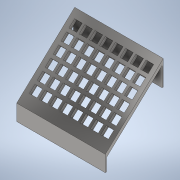
# Autodesk Inventor part: Rejilla_12x12mm
Saved by Autodesk Inventor 2021 (Build 250183000, 183)
## iProperties
Created: 2021-06-27
Part Number: Rejilla_12x12mm
Material: Acero inoxidable
Document SubType Name: Modeling
Designer: artur
Density: 8 g/cm^3
Appearance: Acero - Pulido
Author: artur
Autodesk Inventor part; units mm, degrees
ref_plane "YZ Plane" through (0, 0, 0) normal (1, 0, 0) x (0, 1, 0)
ref_plane "XZ Plane" through (0, 0, 0) normal (0, 1, 0) x (-1, 0, 0)
ref_plane "XY Plane" through (0, 0, 0) normal (0, 0, 1) x (1, 0, 0)
sketch "Boceto3" plane through (0, 0, 0) normal (0, 0, 1) x (1, 0, 0)
  line L0 (118.929, 0) -> (171.1141, 0) construction
  line L1 (0, 0) -> (-79.0081, 0) construction
  line L2 (0, 0) -> (91, 84.6517)
  line L3 (0, 0) -> (0, -24.9684)
  line L4 (0, -24.9684) -> (2, -24.9684)
  line L5 (2, -24.9684) -> (2, -4.9684)
  line L6 (80.5422, 57.5078) -> (86.2007, 57.5078)
  line L7 (91, 84.6517) -> (91, 45.9623)
  line L8 (91, 45.9623) -> (89, 45.9623)
  line L9 (89, 45.9623) -> (89, 75.9623)
  line L10 (2, -4.9684) -> (89, 75.9623)
  dimension "d118" = 137.07
  dimension "d120" = 2
  dimension "d122" = 5
  dimension "d123" = 30
  dimension "d124" = 2
  dimension "d125" = 5
  dimension "d147" = 20
  dimension "d149" = 89
  constraints: 22 end point, 4 horizontal, 2 perpendicular, 2 vertical
  measures "d118" angle of L1 L2
  measures "d120" distance between parallel lines of L5 L3
  measures "d122" distance from line of L2 L9.end
  measures "d123" distance of L8.end L9.end
  measures "d124" distance between parallel lines of L7 L9
  measures "d125" distance from line of L2 L5.end
  measures "d147" distance of L4.end L5.end
  measures "d149" distance between parallel lines of L3 L9
extrude "Extrusión2" add sketch "Boceto3" along normal blind 139
sketch "Boceto7" plane through (0, 0, 0) normal (-0.6811, 0.7322, 0) x (0, 0, 1)
  line L0 (8, 101.2856) -> (20, 101.2856)
  line L1 (20, 101.2856) -> (20, 113.2856)
  line L2 (20, 113.2856) -> (8, 113.2856)
  line L3 (8, 113.2856) -> (8, 101.2856)
  line L4 (0, 124.2856) -> (139, 124.2856) projected
  line L5 (0, 124.2856) -> (0, 0) projected
  line L6 (24, 101.2856) -> (36, 101.2856)
  line L7 (36, 101.2856) -> (36, 113.2856)
  line L8 (36, 113.2856) -> (24, 113.2856)
  line L9 (24, 113.2856) -> (24, 101.2856)
  line L10 (40, 101.2856) -> (52, 101.2856)
  line L11 (52, 101.2856) -> (52, 113.2856)
  line L12 (52, 113.2856) -> (40, 113.2856)
  line L13 (40, 113.2856) -> (40, 101.2856)
  line L14 (56, 101.2856) -> (68, 101.2856)
  line L15 (68, 101.2856) -> (68, 113.2856)
  line L16 (68, 113.2856) -> (56, 113.2856)
  line L17 (56, 113.2856) -> (56, 101.2856)
  line L18 (72, 101.2856) -> (84, 101.2856)
  line L19 (84, 101.2856) -> (84, 113.2856)
  line L20 (84, 113.2856) -> (72, 113.2856)
  line L21 (72, 113.2856) -> (72, 101.2856)
  line L22 (88, 101.2856) -> (100, 101.2856)
  line L23 (100, 101.2856) -> (100, 113.2856)
  line L24 (100, 113.2856) -> (88, 113.2856)
  line L25 (88, 113.2856) -> (88, 101.2856)
  line L26 (104, 101.2856) -> (116, 101.2856)
  line L27 (116, 101.2856) -> (116, 113.2856)
  line L28 (116, 113.2856) -> (104, 113.2856)
  line L29 (104, 113.2856) -> (104, 101.2856)
  line L30 (120, 101.2856) -> (132, 101.2856)
  line L31 (132, 101.2856) -> (132, 113.2856)
  line L32 (132, 113.2856) -> (120, 113.2856)
  line L33 (120, 113.2856) -> (120, 101.2856)
  line L34 (8, 84.2856) -> (20, 84.2856)
  line L35 (8, 96.2856) -> (8, 84.2856)
  line L36 (20, 84.2856) -> (20, 96.2856)
  line L37 (20, 96.2856) -> (8, 96.2856)
  line L38 (24, 96.2856) -> (24, 84.2856)
  line L39 (36, 96.2856) -> (24, 96.2856)
  line L40 (36, 84.2856) -> (36, 96.2856)
  line L41 (24, 84.2856) -> (36, 84.2856)
  line L42 (40, 96.2856) -> (40, 84.2856)
  line L43 (52, 96.2856) -> (40, 96.2856)
  line L44 (40, 84.2856) -> (52, 84.2856)
  line L45 (56, 96.2856) -> (56, 84.2856)
  line L46 (68, 96.2856) -> (56, 96.2856)
  line L47 (56, 84.2856) -> (68, 84.2856)
  line L48 (52, 84.2856) -> (52, 96.2856)
  line L49 (68, 84.2856) -> (68, 96.2856)
  line L50 (72, 96.2856) -> (72, 84.2856)
  line L51 (72, 84.2856) -> (84, 84.2856)
  line L52 (84, 96.2856) -> (72, 96.2856)
  line L53 (84, 84.2856) -> (84, 96.2856)
  line L54 (100, 96.2856) -> (88, 96.2856)
  line L55 (88, 84.2856) -> (100, 84.2856)
  line L56 (88, 96.2856) -> (88, 84.2856)
  line L57 (100, 84.2856) -> (100, 96.2856)
  line L58 (104, 96.2856) -> (104, 84.2856)
  line L59 (116, 96.2856) -> (104, 96.2856)
  line L60 (116, 84.2856) -> (116, 96.2856)
  line L61 (120, 96.2856) -> (120, 84.2856)
  line L62 (132, 84.2856) -> (132, 96.2856)
  line L63 (132, 96.2856) -> (120, 96.2856)
  line L64 (120, 84.2856) -> (132, 84.2856)
  line L65 (104, 84.2856) -> (116, 84.2856)
  line L66 (8, 67.2856) -> (20, 67.2856)
  line L67 (8, 79.2856) -> (8, 67.2856)
  line L68 (20, 67.2856) -> (20, 79.2856)
  line L69 (20, 79.2856) -> (8, 79.2856)
  line L70 (24, 79.2856) -> (24, 67.2856)
  line L71 (36, 79.2856) -> (24, 79.2856)
  line L72 (36, 67.2856) -> (36, 79.2856)
  line L73 (24, 67.2856) -> (36, 67.2856)
  line L74 (40, 79.2856) -> (40, 67.2856)
  line L75 (52, 79.2856) -> (40, 79.2856)
  line L76 (40, 67.2856) -> (52, 67.2856)
  line L77 (56, 79.2856) -> (56, 67.2856)
  line L78 (68, 79.2856) -> (56, 79.2856)
  line L79 (56, 67.2856) -> (68, 67.2856)
  line L80 (52, 67.2856) -> (52, 79.2856)
  line L81 (68, 67.2856) -> (68, 79.2856)
  line L82 (72, 79.2856) -> (72, 67.2856)
  line L83 (72, 67.2856) -> (84, 67.2856)
  line L84 (84, 79.2856) -> (72, 79.2856)
  line L85 (84, 67.2856) -> (84, 79.2856)
  line L86 (100, 79.2856) -> (88, 79.2856)
  line L87 (88, 67.2856) -> (100, 67.2856)
  line L88 (88, 79.2856) -> (88, 67.2856)
  line L89 (100, 67.2856) -> (100, 79.2856)
  line L90 (104, 79.2856) -> (104, 67.2856)
  line L91 (116, 79.2856) -> (104, 79.2856)
  line L92 (116, 67.2856) -> (116, 79.2856)
  line L93 (120, 79.2856) -> (120, 67.2856)
  line L94 (132, 67.2856) -> (132, 79.2856)
  line L95 (132, 79.2856) -> (120, 79.2856)
  line L96 (120, 67.2856) -> (132, 67.2856)
  line L97 (104, 67.2856) -> (116, 67.2856)
  line L98 (8, 50.2856) -> (20, 50.2856)
  line L99 (8, 62.2856) -> (8, 50.2856)
  line L100 (20, 50.2856) -> (20, 62.2856)
  line L101 (20, 62.2856) -> (8, 62.2856)
  line L102 (24, 62.2856) -> (24, 50.2856)
  line L103 (36, 62.2856) -> (24, 62.2856)
  line L104 (36, 50.2856) -> (36, 62.2856)
  line L105 (24, 50.2856) -> (36, 50.2856)
  line L106 (40, 62.2856) -> (40, 50.2856)
  line L107 (52, 62.2856) -> (40, 62.2856)
  line L108 (40, 50.2856) -> (52, 50.2856)
  line L109 (56, 62.2856) -> (56, 50.2856)
  line L110 (68, 62.2856) -> (56, 62.2856)
  line L111 (56, 50.2856) -> (68, 50.2856)
  line L112 (52, 50.2856) -> (52, 62.2856)
  line L113 (68, 50.2856) -> (68, 62.2856)
  line L114 (72, 62.2856) -> (72, 50.2856)
  line L115 (72, 50.2856) -> (84, 50.2856)
  line L116 (84, 62.2856) -> (72, 62.2856)
  line L117 (84, 50.2856) -> (84, 62.2856)
  line L118 (100, 62.2856) -> (88, 62.2856)
  line L119 (88, 50.2856) -> (100, 50.2856)
  line L120 (88, 62.2856) -> (88, 50.2856)
  line L121 (100, 50.2856) -> (100, 62.2856)
  line L122 (104, 62.2856) -> (104, 50.2856)
  line L123 (116, 62.2856) -> (104, 62.2856)
  line L124 (116, 50.2856) -> (116, 62.2856)
  line L125 (120, 62.2856) -> (120, 50.2856)
  line L126 (132, 50.2856) -> (132, 62.2856)
  line L127 (132, 62.2856) -> (120, 62.2856)
  line L128 (120, 50.2856) -> (132, 50.2856)
  line L129 (104, 50.2856) -> (116, 50.2856)
  line L130 (8, 33.2856) -> (20, 33.2856)
  line L131 (8, 45.2856) -> (8, 33.2856)
  line L132 (20, 33.2856) -> (20, 45.2856)
  line L133 (20, 45.2856) -> (8, 45.2856)
  line L134 (24, 45.2856) -> (24, 33.2856)
  line L135 (36, 45.2856) -> (24, 45.2856)
  line L136 (36, 33.2856) -> (36, 45.2856)
  line L137 (24, 33.2856) -> (36, 33.2856)
  line L138 (40, 45.2856) -> (40, 33.2856)
  line L139 (52, 45.2856) -> (40, 45.2856)
  line L140 (40, 33.2856) -> (52, 33.2856)
  line L141 (56, 45.2856) -> (56, 33.2856)
  line L142 (68, 45.2856) -> (56, 45.2856)
  line L143 (56, 33.2856) -> (68, 33.2856)
  line L144 (52, 33.2856) -> (52, 45.2856)
  line L145 (68, 33.2856) -> (68, 45.2856)
  line L146 (72, 45.2856) -> (72, 33.2856)
  line L147 (72, 33.2856) -> (84, 33.2856)
  line L148 (84, 45.2856) -> (72, 45.2856)
  line L149 (84, 33.2856) -> (84, 45.2856)
  line L150 (100, 45.2856) -> (88, 45.2856)
  line L151 (88, 33.2856) -> (100, 33.2856)
  line L152 (88, 45.2856) -> (88, 33.2856)
  line L153 (100, 33.2856) -> (100, 45.2856)
  line L154 (104, 45.2856) -> (104, 33.2856)
  line L155 (116, 45.2856) -> (104, 45.2856)
  line L156 (116, 33.2856) -> (116, 45.2856)
  line L157 (120, 45.2856) -> (120, 33.2856)
  line L158 (132, 33.2856) -> (132, 45.2856)
  line L159 (132, 45.2856) -> (120, 45.2856)
  line L160 (120, 33.2856) -> (132, 33.2856)
  line L161 (104, 33.2856) -> (116, 33.2856)
  line L162 (8, 16.2856) -> (20, 16.2856)
  line L163 (8, 28.2856) -> (8, 16.2856)
  line L164 (20, 16.2856) -> (20, 28.2856)
  line L165 (20, 28.2856) -> (8, 28.2856)
  line L166 (24, 28.2856) -> (24, 16.2856)
  line L167 (36, 28.2856) -> (24, 28.2856)
  line L168 (36, 16.2856) -> (36, 28.2856)
  line L169 (24, 16.2856) -> (36, 16.2856)
  line L170 (40, 28.2856) -> (40, 16.2856)
  line L171 (52, 28.2856) -> (40, 28.2856)
  line L172 (40, 16.2856) -> (52, 16.2856)
  line L173 (56, 28.2856) -> (56, 16.2856)
  line L174 (68, 28.2856) -> (56, 28.2856)
  line L175 (56, 16.2856) -> (68, 16.2856)
  line L176 (52, 16.2856) -> (52, 28.2856)
  line L177 (68, 16.2856) -> (68, 28.2856)
  line L178 (72, 28.2856) -> (72, 16.2856)
  line L179 (72, 16.2856) -> (84, 16.2856)
  line L180 (84, 28.2856) -> (72, 28.2856)
  line L181 (84, 16.2856) -> (84, 28.2856)
  line L182 (100, 28.2856) -> (88, 28.2856)
  line L183 (88, 16.2856) -> (100, 16.2856)
  line L184 (88, 28.2856) -> (88, 16.2856)
  line L185 (100, 16.2856) -> (100, 28.2856)
  line L186 (104, 28.2856) -> (104, 16.2856)
  line L187 (116, 28.2856) -> (104, 28.2856)
  line L188 (116, 16.2856) -> (116, 28.2856)
  line L189 (120, 28.2856) -> (120, 16.2856)
  line L190 (132, 16.2856) -> (132, 28.2856)
  line L191 (132, 28.2856) -> (120, 28.2856)
  line L192 (120, 16.2856) -> (132, 16.2856)
  line L193 (104, 16.2856) -> (116, 16.2856)
  dimension "d126" = 12
  dimension "d127" = 12
  dimension "d128" = 11
  dimension "d129" = 8
  dimension "d132" = 16
  dimension "d139" = 17
  constraints: 384 end point, 2 horizontal, 2 parallel, 1 perpendicular, 1 vertical, 376 other
  measures "d126" distance of L0.end L1.end
  measures "d127" distance of L0.start L0.end
  measures "d128" distance between parallel lines of L4 L2
  measures "d129" distance between parallel lines of L5 L3
  measures "d132" distance of L0.start L6.start
  measures "d139" distance of L0.end L34.end
extrude "Extrusión6" cut sketch "Boceto7" against normal up to surface (5 mm away)
